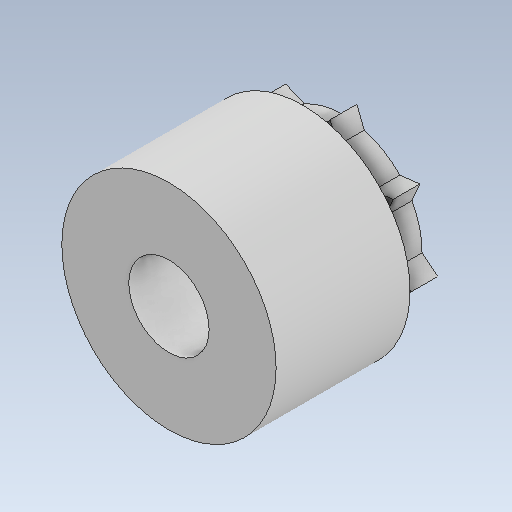
# Autodesk Inventor part: handle_base_potholder
Saved by Autodesk Inventor 2021 (Build 250183000, 183)
## iProperties
Created: 2021-07-05
Part Number: handle_base_potholder
Material: Generic
Document SubType Name: Modeling
Designer: teh18
Density: 1 g/cm^3
Appearance: Default
Author: teh18
Autodesk Inventor part; units mm, degrees
ref_plane "YZ Plane" through (0, 0, 0) normal (1, 0, 0) x (0, 1, 0)
ref_plane "XZ Plane" through (0, 0, 0) normal (0, 1, 0) x (-1, 0, 0)
ref_plane "XY Plane" through (0, 0, 0) normal (0, 0, 1) x (1, 0, 0)
sketch "Sketch1" plane through (0, 0, 0) normal (0, 0, 1) x (1, 0, 0)
  circle A0 centre (0, 0) radius 8 projected
  arc A1 (-4.1006, 4.2421) -> (-5.6821, 1.5887) centre (0, 0) ccw projected
  line L0 (-5.6821, 1.5887) -> (-7.0798, 1.0323) projected
  line L1 (-7.0798, 1.0323) -> (-5.8992, 0.1) projected
  arc A2 (-5.8992, 0.1) -> (-5.1412, -2.8945) centre (0, 0) ccw projected
  line L2 (-5.1412, -2.8945) -> (-5.7362, -4.2762) projected
  line L3 (-5.7362, -4.2762) -> (-4.2421, -4.1006) projected
  arc A3 (-4.2421, -4.1006) -> (-1.5887, -5.6821) centre (0, 0) ccw projected
  line L4 (-1.5887, -5.6821) -> (-1.0323, -7.0798) projected
  line L5 (-1.0323, -7.0798) -> (-0.1, -5.8992) projected
  arc A4 (-0.1, -5.8992) -> (2.8945, -5.1412) centre (0, 0) ccw projected
  line L6 (2.8945, -5.1412) -> (4.2762, -5.7362) projected
  line L7 (4.2762, -5.7362) -> (4.1006, -4.2421) projected
  arc A5 (4.1006, -4.2421) -> (5.6821, -1.5887) centre (0, 0) ccw projected
  line L8 (5.6821, -1.5887) -> (7.0798, -1.0323) projected
  line L9 (7.0798, -1.0323) -> (5.8992, -0.1) projected
  arc A6 (5.8992, -0.1) -> (5.1412, 2.8945) centre (0, 0) ccw projected
  line L10 (5.1412, 2.8945) -> (5.7362, 4.2762) projected
  line L11 (5.7362, 4.2762) -> (4.2421, 4.1006) projected
  arc A7 (4.2421, 4.1006) -> (1.5887, 5.6821) centre (0, 0) ccw projected
  line L12 (1.5887, 5.6821) -> (1.0323, 7.0798) projected
  line L13 (1.0323, 7.0798) -> (0.1, 5.8992) projected
  arc A8 (0.1, 5.8992) -> (-2.8945, 5.1412) centre (0, 0) ccw projected
  line L14 (-2.8945, 5.1412) -> (-4.2762, 5.7362) projected
  line L15 (-4.2762, 5.7362) -> (-4.1006, 4.2421) projected
  line L16 (7.2794, -1.0614) -> (5.7655, -1.664) projected
  arc A9 (4.2066, -4.2796) -> (5.7655, -1.664) centre (0, 0) ccw projected
  line L17 (4.2066, -4.2796) -> (4.3968, -5.8979) projected
  line L18 (4.3968, -5.8979) -> (2.9002, -5.2535) projected
  arc A10 (-0.0517, -6.0006) -> (2.9002, -5.2535) centre (0, 0) ccw projected
  line L19 (-0.0517, -6.0006) -> (-1.0614, -7.2794) projected
  line L20 (-1.0614, -7.2794) -> (-1.664, -5.7655) projected
  arc A11 (-4.2796, -4.2066) -> (-1.664, -5.7655) centre (0, 0) ccw projected
  line L21 (-4.2796, -4.2066) -> (-5.8979, -4.3968) projected
  line L22 (-5.8979, -4.3968) -> (-5.2535, -2.9002) projected
  arc A12 (-6.0006, 0.0517) -> (-5.2535, -2.9002) centre (0, 0) ccw projected
  line L23 (-6.0006, 0.0517) -> (-7.2794, 1.0614) projected
  line L24 (-7.2794, 1.0614) -> (-5.7655, 1.664) projected
  arc A13 (-4.2066, 4.2796) -> (-5.7655, 1.664) centre (0, 0) ccw projected
  line L25 (-4.2066, 4.2796) -> (-4.3968, 5.8979) projected
  line L26 (-4.3968, 5.8979) -> (-2.9002, 5.2535) projected
  arc A14 (0.0517, 6.0006) -> (-2.9002, 5.2535) centre (0, 0) ccw projected
  line L27 (0.0517, 6.0006) -> (1.0614, 7.2794) projected
  line L28 (1.0614, 7.2794) -> (1.664, 5.7655) projected
  arc A15 (4.2796, 4.2066) -> (1.664, 5.7655) centre (0, 0) ccw projected
  line L29 (4.2796, 4.2066) -> (5.8979, 4.3968) projected
  line L30 (5.8979, 4.3968) -> (5.2535, 2.9002) projected
  arc A16 (6.0006, -0.0517) -> (5.2535, 2.9002) centre (0, 0) ccw projected
  line L31 (6.0006, -0.0517) -> (7.2794, -1.0614) projected
  circle A17 centre (0, 0) radius 18 projected
  point P0 (0, 0)
extrude "Extrusion1" add sketch "Sketch1" against normal blind 2 contours L15 L14 A8 L13 L12 A7 L11 L10 A6 L9 L8 A5 L7 L6 A4 L5 L4 A3 L3 L2 A2 L1 L0 A1
sketch "Sketch2" plane through (0, 0, 0) normal (0, 0, 1) x (1, 0, 0)
  line L0 (7.2794, -1.0614) -> (5.7655, -1.664) projected
  arc A0 (4.2066, -4.2796) -> (5.7655, -1.664) centre (0, 0) ccw projected
  line L1 (4.2066, -4.2796) -> (4.3968, -5.8979) projected
  line L2 (4.3968, -5.8979) -> (2.9002, -5.2535) projected
  arc A1 (-0.0517, -6.0006) -> (2.9002, -5.2535) centre (0, 0) ccw projected
  line L3 (-0.0517, -6.0006) -> (-1.0614, -7.2794) projected
  line L4 (-1.0614, -7.2794) -> (-1.664, -5.7655) projected
  arc A2 (-4.2796, -4.2066) -> (-1.664, -5.7655) centre (0, 0) ccw projected
  line L5 (-4.2796, -4.2066) -> (-5.8979, -4.3968) projected
  line L6 (-5.8979, -4.3968) -> (-5.2535, -2.9002) projected
  arc A3 (-6.0006, 0.0517) -> (-5.2535, -2.9002) centre (0, 0) ccw projected
  line L7 (-6.0006, 0.0517) -> (-7.2794, 1.0614) projected
  line L8 (-7.2794, 1.0614) -> (-5.7655, 1.664) projected
  arc A4 (-4.2066, 4.2796) -> (-5.7655, 1.664) centre (0, 0) ccw projected
  line L9 (-4.2066, 4.2796) -> (-4.3968, 5.8979) projected
  line L10 (-4.3968, 5.8979) -> (-2.9002, 5.2535) projected
  arc A5 (0.0517, 6.0006) -> (-2.9002, 5.2535) centre (0, 0) ccw projected
  line L11 (0.0517, 6.0006) -> (1.0614, 7.2794) projected
  line L12 (1.0614, 7.2794) -> (1.664, 5.7655) projected
  arc A6 (4.2796, 4.2066) -> (1.664, 5.7655) centre (0, 0) ccw projected
  line L13 (4.2796, 4.2066) -> (5.8979, 4.3968) projected
  line L14 (5.8979, 4.3968) -> (5.2535, 2.9002) projected
  arc A7 (6.0006, -0.0517) -> (5.2535, 2.9002) centre (0, 0) ccw projected
  line L15 (6.0006, -0.0517) -> (7.2794, -1.0614) projected
  circle A8 centre (0, 0) radius 3
  line L16 (-3, 0.5) -> (3, 0.5)
  line L17 (3, 0.5) -> (3, -0.5)
  line L18 (3, -0.5) -> (-3, -0.5)
  line L19 (-3, -0.5) -> (-3, 0.5)
  line L20 (-3, 0.5) -> (3, -0.5) construction
  line L21 (3, 0.5) -> (-3, -0.5) construction
  circle A9 centre (0, 0) radius 18 projected
  point P0 (0, 0)
  point P1 (-3, 0)
  point P2 (-2.958, 0.5)
  point P3 (2.958, 0.5)
  point P4 (3, 0)
  point P5 (2.958, -0.5)
  point P6 (-2.958, -0.5)
  dimension "d2" = 6
  dimension "d3" = 6
  dimension "d4" = 1
  constraints: 12 end point, 2 midpoint, 2 parallel, 1 centre point, 1 horizontal, 1 perpendicular
  measures "d2" diameter of A8
  measures "d3" distance of L17.end L18.end
  measures "d4" distance of L16.end L17.end
extrude "Extrusion2" add sketch "Sketch2" along normal blind 1 contours A8 L18 L16
sketch "Sketch3" plane through (0, 0, 1) normal (0, 0, 1) x (1, 0, 0)
  circle A0 centre (0, 0) radius 8 projected
  arc A1 (-2.958, -0.5) -> (2.958, -0.5) centre (0, 0) ccw projected
  line L0 (-2.958, -0.5) -> (2.958, -0.5) projected
  line L1 (2.958, 0.5) -> (-2.958, 0.5) projected
  arc A2 (2.958, 0.5) -> (-2.958, 0.5) centre (0, 0) ccw projected
  circle A3 centre (0, 0) radius 3
  point P0 (0, 0)
  point P1 (-2.958, -0.5)
  point P2 (-2.958, 0.5)
  point P3 (2.958, 0.5)
  point P4 (2.958, -0.5)
  constraints: 1 centre point, 1 coincident
extrude "Extrusion3" add sketch "Sketch3" along normal blind 10
body "Solid1"
